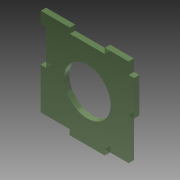
# Autodesk Inventor part: Side B
Saved by Autodesk Inventor 2014 SP2 (Build 180246200, 246)
## iProperties
Created: 2014-11-21
Part Number: Side B
Material: Generic
Document SubType Name: Modeling
Designer: JLM
Density: 1 g/cm^3
Appearance: Default
Author: JLM
Autodesk Inventor part; units mm, degrees
ref_plane "YZ Plane" through (0, 0, 0) normal (1, 0, 0) x (0, 1, 0)
ref_plane "XZ Plane" through (0, 0, 0) normal (0, 1, 0) x (-1, 0, 0)
ref_plane "XY Plane" through (0, 0, 0) normal (0, 0, 1) x (1, 0, 0)
sketch "Sketch1" plane through (0, 0, 0) normal (0, 0, 1) x (1, 0, 0)
  line L0 (-25.4, -25.4) -> (25.4, -25.4)
  line L1 (25.4, -25.4) -> (25.4, 25.4)
  line L2 (25.4, 25.4) -> (-25.4, 25.4)
  line L3 (-25.4, 25.4) -> (-25.4, -25.4)
  line L4 (-25.4, -25.4) -> (25.4, 25.4) construction
  line L5 (25.4, -25.4) -> (-25.4, 25.4) construction
  point P0 (0, 0)
  dimension "d0" = 50.8
  dimension "d1" = 50.8
  constraints: 12 end point, 2 midpoint, 2 parallel, 1 horizontal, 1 perpendicular
  measures "d0" distance of L2.end L1.end
  measures "d1" distance of L1.end L0.end
extrude "Extrusion1" add sketch "Sketch1" against normal blind 2.921
sketch "Sketch4" plane through (0, 0, 0) normal (0, 0, 1) x (1, 0, 0)
  line L0 (25.4, -22.4923) -> (9.525, -22.4923)
  line L1 (9.525, -22.4923) -> (9.525, -25.4133)
  line L2 (9.525, -25.4133) -> (25.4, -25.4133)
  line L3 (25.4, -25.4133) -> (25.4, -22.4923)
  line L4 (-25.4, -25.4) -> (-9.525, -25.4)
  line L5 (-9.525, -25.4) -> (-9.525, -22.479)
  line L6 (-9.525, -22.479) -> (-25.4, -22.479)
  line L7 (-25.4, -22.479) -> (-25.4, -25.4)
  line L8 (25.4, -25.4) -> (25.4, 25.4) projected
  line L9 (25.4, 25.4) -> (-25.4, 25.4) projected
  line L10 (-25.4, 25.4) -> (-25.4, -25.4) projected
  line L11 (-25.4, 19.05) -> (-22.479, 19.05)
  line L12 (-22.479, 19.05) -> (-22.479, 0)
  line L13 (-22.479, 0) -> (-25.4, 0)
  line L14 (-25.4, 0) -> (-25.4, 19.05)
  line L15 (25.4, 19.05) -> (22.479, 19.05)
  line L16 (22.479, 0) -> (25.4, 0)
  line L17 (25.4, 0) -> (25.4, 19.05)
  line L18 (-9.525, 25.4) -> (9.525, 25.4)
  line L19 (9.525, 25.4) -> (9.525, 22.479)
  line L20 (9.525, 22.479) -> (-9.525, 22.479)
  line L21 (-9.525, 22.479) -> (-9.525, 25.4)
  line L22 (-25.4, -25.4) -> (25.4, -25.4) projected
  line L23 (22.479, 19.05) -> (22.479, 25.4)
  line L24 (22.479, 0) -> (22.479, -25.4)
  point P0 (0, 0)
  dimension "d12" = 15.875
  dimension "d13" = 2.921
  dimension "d16" = 2.921
  dimension "d37" = 9.525
  dimension "d38" = 15.875
  dimension "d39" = 9.525
  dimension "d40" = 2.921
  dimension "d41" = 2.921
  dimension "d42" = 19.05
  dimension "d44" = 2.921
  dimension "d45" = 19.05
  dimension "d46" = 15.875
  dimension "d50" = 25.4
  dimension "d52" = 50.8
  dimension "d53" = 50.8
  dimension "d54" = 25.4
  dimension "d55" = 44.958
  dimension "d56" = 44.958
  constraints: 42 end point, 9 parallel, 6 perpendicular, 5 horizontal, 5 point on line, 2 collinear
  measures "d12" distance of L2.end L1.end
  measures "d13" distance of L1.end L0.end
  measures "d16" distance of L4.end L5.end
  measures "d37" distance from line of point (0, 0) L5
  measures "d38" distance of L4.start L4.end
  measures "d39" distance from line of point (0, 0) L1
  measures "d40" distance of L11.start L11.end
  measures "d41" distance of L15.start L15.end
  measures "d42" distance of L11.end L12.end
  measures "d44" distance of L20.end L18.start
  measures "d45" distance of L19.end L20.end
  measures "d46" distance between parallel lines of L10 L21
  measures "d50" distance between parallel lines of L4 L13
  measures "d52" distance between parallel lines of L8 L10
  measures "d53" distance between parallel lines of L22 L9
  measures "d54" distance between parallel lines of L22 L16
  measures "d55" distance between parallel lines of L6 L20
  measures "d56" distance between parallel lines of L24 L12
extrude "Extrusion5" cut sketch "Sketch4" against normal blind 25.4 contours L3 L22 L24 L0 | L0 L24 L16 L8 | L24 L22 L1 L0 | L3 L2 L1 L22 | L15 L23 L9 L8 | L4 L7 L6 L5 | L19 L20 L21 L9 | L10 L11 L12 L13
hole "Hole1" at (0, 0, 0) direction (0, 0, -1) diameter 25.4 end through all
equation "\"d12\" = d38"
equation "\"d13\" = d16"
equation "\"d38\" = -d37 + 0.5 * d0"
equation "\"d39\" = d37"
equation "\"d40\" = d16"
equation "\"d41\" = d16"
equation "\"d42\" = 2 * d37"
equation "\"d44\" = d16"
equation "\"d45\" = d42"
equation "\"d46\" = d38"
equation "\"d54\" = d50"
equation "\"d48\" = 0.5 * d0"
body "Solid1"
